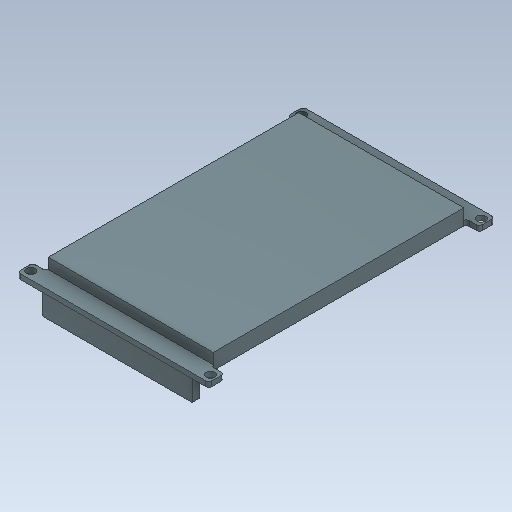
# Autodesk Inventor part: TouchLCD
Saved by Autodesk Inventor 2020 (Build 240168000, 168)
## iProperties
Created: 2020-04-08
Part Number: TouchLCD
Material: Lead
Document SubType Name: Modeling
Designer: Samuele
Density: 11.34 g/cm^3
Appearance: Lead
Author: Samuele
Autodesk Inventor part; units mm, degrees
ref_plane "YZ Plane" through (0, 0, 0) normal (1, 0, 0) x (0, 1, 0)
ref_plane "XZ Plane" through (0, 0, 0) normal (0, 1, 0) x (-1, 0, 0)
ref_plane "XY Plane" through (0, 0, 0) normal (0, 0, 1) x (1, 0, 0)
sketch "Sketch1" plane through (0, 0, 0) normal (0, 1, 0) x (-1, 0, 0)
  line L0 (0, 0) -> (56, 0)
  line L1 (56, -6.2) -> (56, -90.8)
  line L2 (56, -97) -> (0, -97)
  line L3 (0, -90.8) -> (0, -6.2)
  line L4 (0, 0) -> (-3.5, 0)
  line L5 (-4.5, -1) -> (-4.5, -4.2)
  line L6 (-3.5, -5.2) -> (-1, -5.2)
  line L7 (28, 0) -> (28, -97)
  circle A0 centre (-2.5, -2.6) radius 1.5
  arc A1 (-3.5, 0) -> (-4.5, -1) centre (-3.5, -1) ccw
  arc A2 (-4.5, -4.2) -> (-3.5, -5.2) centre (-3.5, -4.2) ccw
  arc A3 (0, -6.2) -> (-1, -5.2) centre (-1, -6.2) ccw
  line L8 (56, 0) -> (59.5, 0)
  line L9 (60.5, -1) -> (60.5, -4.2)
  line L10 (59.5, -5.2) -> (57, -5.2)
  circle A4 centre (58.5, -2.6) radius 1.5
  arc A5 (60.5, -1) -> (59.5, 0) centre (59.5, -1) ccw
  arc A6 (59.5, -5.2) -> (60.5, -4.2) centre (59.5, -4.2) ccw
  arc A7 (57, -5.2) -> (56, -6.2) centre (57, -6.2) ccw
  line L11 (56, -48.5) -> (0, -48.5)
  line L12 (0, -97) -> (-3.5, -97)
  line L13 (-4.5, -96) -> (-4.5, -92.8)
  line L14 (-3.5, -91.8) -> (-1, -91.8)
  circle A8 centre (-2.5, -94.4) radius 1.5
  arc A9 (-4.5, -96) -> (-3.5, -97) centre (-3.5, -96) ccw
  arc A10 (-3.5, -91.8) -> (-4.5, -92.8) centre (-3.5, -92.8) ccw
  arc A11 (-1, -91.8) -> (0, -90.8) centre (-1, -90.8) ccw
  arc A12 (56, -90.8) -> (57, -91.8) centre (57, -90.8) ccw
  line L15 (59.5, -91.8) -> (57, -91.8)
  line L16 (56, -97) -> (59.5, -97)
  circle A13 centre (58.5, -94.4) radius 1.5
  arc A14 (60.5, -92.8) -> (59.5, -91.8) centre (59.5, -92.8) ccw
  line L17 (60.5, -96) -> (60.5, -92.8)
  arc A15 (59.5, -97) -> (60.5, -96) centre (59.5, -96) ccw
  point P0 (-4.5, 0)
  point P1 (-4.5, -5.2)
  point P2 (0, -5.2)
  point P3 (60.5, 0)
  point P4 (60.5, -5.2)
  point P5 (56, -5.2)
  point P6 (-4.5, -97)
  point P7 (-4.5, -91.8)
  point P8 (0, -91.8)
  point P9 (56, -91.8)
  point P10 (60.5, -91.8)
  point P11 (60.5, -97)
  dimension "d0" = 56
  dimension "d1" = 97
  dimension "d2" = 4.5
  dimension "d3" = 5.2
  dimension "d10" = 1
  dimension "d11" = 1
  dimension "d12" = 2
  dimension "d13" = 2.6
  dimension "d14" = 3
  dimension "d15" = 56
  constraints: 39 symmetric about line, 36 end point, 24 point on circle, 22 point on line, 16 centre point, 6 tangent, 4 midpoint, 3 horizontal, 3 perpendicular, 2 parallel, 1 equal radius, 12 other
  measures "d0" distance of L2.start L2.end
  measures "d1" distance of L0.end L2.start
  measures "d2" distance of L0.start point (-4.5, 0)
  measures "d3" distance of point (-4.5, 0) point (-4.5, -5.2)
  measures "d10" radius of A1
  measures "d11" radius of A3
  measures "d12" distance from line of L5 A0.centre
  measures "d13" distance from line of L6 A0.centre
  measures "d14" diameter of A0
  measures "d15" distance between parallel lines of L3 L1
extrude "Vetronite" add sketch "Sketch1" along normal blind 1.7
sketch "Sketch2" plane through (0, 1.7, 0) normal (0, 1, 0) x (1, 0, 0)
  line L0 (-59.5, 0) -> (3.5, 0) projected
  line L1 (-28, 0) -> (-28, 97)
  line L2 (3.5, 97) -> (-59.5, 97) projected
  line L3 (-56, 90.8) -> (-56, 6.2) projected
  line L4 (-56, 48.5) -> (0, 48.5)
  line L5 (0, 6.2) -> (0, 90.8) projected
  line L6 (-56, 6) -> (0, 6)
  line L7 (0, 6) -> (0, 91)
  line L8 (0, 91) -> (-56, 91)
  line L9 (-56, 91) -> (-56, 6)
  point P0 (0, 0)
  point P1 (-56, 6.2)
  dimension "d16" = 85
  dimension "d17" = 56
  constraints: 12 end point, 4 midpoint, 2 parallel, 1 horizontal, 1 perpendicular, 2 other
  measures "d16" distance of L8.end L6.start
  measures "d17" distance of L6.start L6.end
extrude "Display" add sketch "Sketch2" along normal blind 3.6
sketch "Sketch3" plane through (0, 0, 0) normal (0, -1, 0) x (1, 0, 0)
  line L0 (-53.3, -4) -> (-2.7, -4)
  line L1 (-2.7, -4) -> (-2.7, -1.5)
  line L2 (-2.7, -1.5) -> (-53.3, -1.5)
  line L3 (-53.3, -1.5) -> (-53.3, -4)
  line L4 (-59.5, 0) -> (3.5, 0) projected
  line L5 (3.5, -97) -> (-59.5, -97) projected
  line L6 (-28, -97) -> (-28, 0)
  line L7 (-59.5, 0) -> (3.5, 0) projected
  point P0 (0, 0)
  dimension "d20" = 50.6
  dimension "d21" = 2.5
  dimension "d22" = 1.5
  constraints: 10 end point, 2 midpoint, 2 parallel, 1 horizontal, 1 perpendicular, 1 other
  measures "d20" distance of L2.end L1.end
  measures "d21" distance of L1.end L0.end
  measures "d22" distance between parallel lines of L2 L4
extrude "Pin" add sketch "Sketch3" along normal blind 8.5
sketch "Sketch4" plane through (0, 0, 0) normal (0, -1, 0) x (1, 0, 0)
  line L0 (-5, -82) -> (-21, -82)
  line L1 (-21, -82) -> (-21, -68)
  line L2 (-21, -68) -> (-5, -68)
  line L3 (-5, -68) -> (-5, -82)
  line L4 (-50, -69) -> (-38, -69)
  line L5 (-38, -69) -> (-38, -57)
  line L6 (-38, -57) -> (-50, -57)
  line L7 (-50, -57) -> (-50, -69)
  line L8 (-36, -69) -> (-24, -69)
  line L9 (-24, -69) -> (-24, -57)
  line L10 (-24, -57) -> (-36, -57)
  line L11 (-36, -57) -> (-36, -69)
  line L12 (-43, -40) -> (-13, -40)
  line L13 (-13, -40) -> (-13, -24)
  line L14 (-13, -24) -> (-43, -24)
  line L15 (-43, -24) -> (-43, -40)
  line L16 (3.5, -97) -> (-59.5, -97) projected
  line L17 (0, -6.2) -> (0, -90.8) projected
  line L18 (-56, -90.8) -> (-56, -6.2) projected
  point P0 (0, 0)
  dimension "d25" = 16
  dimension "d26" = 14
  dimension "d27" = 12
  dimension "d28" = 12
  dimension "d29" = 12
  dimension "d30" = 12
  dimension "d31" = 30
  dimension "d32" = 16
  dimension "d33" = 15
  dimension "d34" = 5
  dimension "d35" = 28
  dimension "d36" = 6
  dimension "d37" = 2
  dimension "d38" = 57
  dimension "d40" = 13
  constraints: 32 end point, 8 parallel, 4 horizontal, 4 perpendicular, 1 collinear
  measures "d25" distance of L1.end L2.end
  measures "d26" distance of L0.end L1.end
  measures "d27" distance of L6.end L5.end
  measures "d28" distance of L5.end L4.end
  measures "d29" distance of L10.end L9.end
  measures "d30" distance of L9.end L8.end
  measures "d31" distance of L14.end L13.end
  measures "d32" distance of L13.end L12.end
  measures "d33" distance between parallel lines of L16 L0
  measures "d34" distance between parallel lines of L17 L3
  measures "d35" distance between parallel lines of L4 L16
  measures "d36" distance between parallel lines of L18 L7
  measures "d37" distance between parallel lines of L5 L11
  measures "d38" distance between parallel lines of L12 L16
  measures "d40" distance between parallel lines of L18 L15
extrude "Componenti" add sketch "Sketch4" along normal blind 2.5
draft "ScreenCables" angle 80 pull direction (0, -1, 0) faces at (-23, -0.8333, -24) fixed edges at (-28, 0, -24)
body "Solid1"
